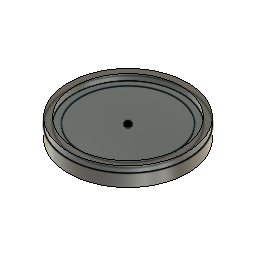
pogo_rig_rev2_v19 (Autodesk Fusion 360 archive; units mm, degrees)
design "PCB sizing rev G"
Autodesk Fusion 360 part; units mm, degrees
sketch "Sketch1" plane through (0, 0, 0) normal (0, 0, 1) x (1, 0, 0)
  circle A0 centre (0, 0) radius 8.5
  circle A1 centre (0, 0) radius 7.5
  circle A2 centre (0, 0) radius 9.5
  dimension "d1" = 17
  dimension "d2" = 15
  dimension "d3" = 19
  constraint coincident A0.centre A1.centre
  constraint concentric A0 A1
  constraint concentric A1 A2
  measures "d1" diameter of A0
  measures "d2" diameter of A1
  measures "d3" diameter of A2
extrude "Extrude1" add sketch "Sketch1" against normal blind 2 contours A0 | A1 | A2
extrude "Extrude2" add sketch "Sketch1" along normal blind 1 contours A2
